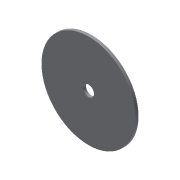
# Autodesk Inventor part: SpoolGuard
Saved by Autodesk Inventor 2015 (Build 190159000, 159)
## iProperties
Created: 2015-03-09
Part Number: SpoolGuard
Material: Generic
Document SubType Name: Modeling
Designer: Jaden
Density: 1 g/cm^3
Appearance: Default
Author: Jaden
Autodesk Inventor part; units mm, degrees
ref_plane "YZ Plane" through (0, 0, 0) normal (1, 0, 0) x (0, 1, 0)
ref_plane "XZ Plane" through (0, 0, 0) normal (0, 1, 0) x (-1, 0, 0)
ref_plane "XY Plane" through (0, 0, 0) normal (0, 0, 1) x (1, 0, 0)
sketch "Sketch1" plane through (0, 0, 0) normal (0, 0, 1) x (1, 0, 0)
  circle A0 centre (0, 0) radius 41.275
  dimension "d10" = 82.55
  constraints: 1 centre point
  measures "d10" diameter of A0
extrude "Extrusion1" add sketch "Sketch1" along normal blind 2.54
hole "Hole1" at (0, 0, 2.54) direction (0, 0, -1) diameter 9.525 end through all
body "Solid1"
